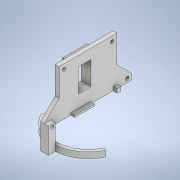
# Autodesk Inventor part: StaticGripper
Saved by Autodesk Inventor 2020 (Build 240168000, 168)
## iProperties
Created: 2023-01-18
Part Number: StaticGripper
Material: Generic
Document SubType Name: Modeling
Designer: legoo
Density: 1 g/cm^3
Appearance: Default
Author: legoo
## iProperties of the stored document _3DPrint.ipt
Created: 2023-01-18
Part Number: _3DPrint
Material: Generic
Document SubType Name: Modeling
Designer: legoo
Density: 1 g/cm^3
Appearance: Default
Author: legoo
Autodesk Inventor part; units mm, degrees
ref_plane "YZ Plane" through (0, 0, 0) normal (1, 0, 0) x (0, 1, 0)
ref_plane "XZ Plane" through (0, 0, 0) normal (0, 1, 0) x (-1, 0, 0)
ref_plane "XY Plane" through (0, 0, 0) normal (0, 0, 1) x (1, 0, 0)
sketch "Sketch1" plane through (0, 0, 0) normal (0, 1, 0) x (-1, 0, 0)
  line L0 (32.6452, 15.2227) -> (29.9263, 13.9549)
  line L1 (-29.9263, 13.9549) -> (-32.6452, 15.2227)
  line L2 (36.02, 0) -> (-36.02, 0) construction
  arc A0 (29.9263, 13.9549) -> (-29.9263, 13.9549) centre (0, 0) ccw
  arc A1 (32.6452, 15.2227) -> (-32.6452, 15.2227) centre (0, 0) ccw
  dimension "d2" = 25
  dimension "d3" = 25
  constraints: 6 end point, 4 point on circle, 2 centre point, 1 coincident, 1 horizontal
  measures "d2" angle of L0 L2
  measures "d3" angle of L2 L1
extrude "Extrusion1" add sketch "Sketch1" along normal blind 6
sketch "Sketch2" plane through (0, 0, 0) normal (0, -1, 0) x (1, 0, 0)
  arc A0 (32.6452, 15.2227) -> (-32.6452, 15.2227) centre (0, 0) ccw projected
  line L0 (2, 35.9644) -> (2, 42.9644)
  line L1 (2, 42.9644) -> (-2, 42.9644)
  line L2 (-2, 42.9644) -> (-2, 35.9644)
  dimension "d6" = 2
  dimension "d7" = 2
  dimension "d8" = 7
  constraints: 6 end point, 2 perpendicular, 2 point on circle, 1 vertical
  measures "d6" distance from line of point (0, 0) L0
  measures "d7" distance from line of point (0, 0) L2
  measures "d8" distance of L0.start L0.end
extrude "Extrusion2" add sketch "Sketch2" against normal blind 26
sketch "Sketch3" plane through (-2, 0, 35.9644) normal (-1, 0, 0) x (0, 0, 1)
  line L0 (7, 0) -> (7, 26) projected
  line L1 (7, 20) -> (-82.04, 20)
  line L2 (-82.04, 20) -> (-82.04, 26)
  line L3 (-82.04, 26) -> (-67.04, 41)
  line L4 (-67.04, 41) -> (-67.04, 69)
  line L5 (-67.04, 69) -> (-8, 69)
  line L6 (-8, 69) -> (-8, 41)
  line L7 (-8, 41) -> (7, 26)
  line L8 (-40.52, 59) -> (-27.52, 59)
  line L9 (-27.52, 59) -> (-27.52, 35)
  line L10 (-27.52, 35) -> (-40.52, 35)
  line L11 (-40.52, 35) -> (-40.52, 59)
  line L12 (7, 0) -> (0, 0) projected
  point P0 (-35.9644, 0)
  dimension "d11" = 15
  dimension "d12" = 15
  dimension "d13" = 89.04
  dimension "d14" = 24
  dimension "d15" = 13
  dimension "d16" = 19.52
  dimension "d17" = 10
  dimension "d18" = 15
  dimension "d19" = 15
  dimension "d20" = 15
  dimension "d21" = 20
  dimension "d22" = 6
  constraints: 22 end point, 4 perpendicular, 3 parallel, 2 horizontal, 1 point on line
  measures "d11" horizontal distance of L6.end L0.end
  measures "d12" horizontal distance of L3.end L2.end
  measures "d13" distance between parallel lines of L2 L0
  measures "d14" distance of L8.end L9.end
  measures "d15" distance of L8.start L8.end
  measures "d16" distance between parallel lines of L6 L9
  measures "d17" distance between parallel lines of L8 L5
  measures "d18" distance between parallel lines of L1 L10
  measures "d19" horizontal distance of L2.end L3.end
  measures "d20" horizontal distance of L0.end L6.end
  measures "d21" distance between parallel lines of L12 L1
  measures "d22" distance of L1.end L2.end
extrude "Extrusion3" add sketch "Sketch3" along normal blind 4
sketch "Sketch4" plane through (-6, 0, 35.9644) normal (-1, 0, 0) x (0, 0, 1)
  line L0 (-40.52, 35) -> (-40.52, 59) projected
  line L1 (-27.52, 35) -> (-40.52, 35) projected
  line L2 (-27.52, 59) -> (-27.52, 35) projected
  line L3 (-40.52, 59) -> (-27.52, 59) projected
  line L4 (-46.52, 29) -> (-46.52, 65)
  line L5 (-46.52, 65) -> (-21.52, 65)
  line L6 (-21.52, 65) -> (-21.52, 29)
  line L7 (-21.52, 29) -> (-46.52, 29)
  point P0 (-35.9644, 0)
  dimension "d49" = 6
  constraints: 8 end point, 3 other
  measures "d49" distance between parallel lines of L0 L4
extrude "Extrusion4" add sketch "Sketch4" along normal blind 6
sketch "Sketch5" plane through (-2, 20, -46.0756) normal (0, -1, 0) x (1, 0, 0)
  line L0 (0, 82.04) -> (0, 89.04) projected
  line L1 (0, 82.04) -> (0, 89.04)
  line L2 (0, 89.04) -> (-4, 89.04) projected
  line L3 (0, 89.04) -> (-4, 89.04)
  line L4 (-4, 89.04) -> (-4, 81.54)
  line L5 (-4, 89.04) -> (-4, 74.04) projected
  arc A0 (0, 82.04) -> (-30.6452, 61.2983) centre (2, 46.0756) ccw projected
  point P0 (-4, 81.5923)
  constraints: 6 end point, 2 collinear, 1 midpoint
extrude "Extrusion5" add sketch "Sketch5" along normal up to surface (20 mm away)
sketch "Sketch6" plane through (-2, 0, 35.9644) normal (1, 0, 0) x (0, 0, -1)
  circle A0 centre (77.54, 24) radius 1.75
  circle A1 centre (62.04, 64) radius 1.75
  circle A2 centre (13, 64) radius 1.75
  line L0 (8, 69) -> (67.04, 69) projected
  line L1 (67.04, 69) -> (67.04, 41) projected
  line L2 (8, 41) -> (8, 69) projected
  line L3 (82.04, 20) -> (0, 20) projected
  line L4 (82.04, 26) -> (82.04, 20) projected
  point P0 (35.9644, 0)
  dimension "d36" = 3.5
  dimension "d37" = 3.5
  dimension "d38" = 3.5
  dimension "d40" = 5
  dimension "d41" = 5
  dimension "d42" = 5
  dimension "d43" = 5
  dimension "d44" = 4
  dimension "d45" = 4.5
  constraints: 3 centre point
  measures "d36" diameter of A1
  measures "d37" diameter of A2
  measures "d38" diameter of A0
  measures "d40" distance from line of A1.centre L0
  measures "d41" distance from line of L1 A1.centre
  measures "d42" distance from line of L2 A2.centre
  measures "d43" distance from line of A2.centre L0
  measures "d44" distance from line of L3 A0.centre
  measures "d45" distance from line of L4 A0.centre
extrude "Extrusion6" cut sketch "Sketch6" against normal blind 6
sketch "Sketch7" plane through (2, 0, 42.9644) normal (1, 0, 0) x (0, 0, -1)
  circle A0 centre (4, 23) radius 1.75
  line L0 (0, 0) -> (0, 26) projected
  line L1 (0, 26) -> (7, 26) projected
  point P0 (42.9644, 0)
  dimension "d50" = 3.5
  dimension "d51" = 4
  dimension "d52" = 3
  constraints: 1 centre point
  measures "d50" diameter of A0
  measures "d51" distance from line of L0 A0.centre
  measures "d52" distance from line of L1 A0.centre
extrude "Extrusion7" cut sketch "Sketch7" against normal through all
sketch "Sketch8" plane through (-2, 0, 35.9644) normal (1, 0, 0) x (0, 0, -1)
  line L0 (82.04, 20) -> (0, 20) projected
  line L1 (20, 22) -> (40, 22)
  line L2 (40, 22) -> (40, 20)
  line L3 (40, 20) -> (20, 20)
  line L4 (20, 20) -> (20, 22)
  line L5 (0, 6) -> (0, 26) projected
  line L6 (67.04, 20) -> (63.04, 20)
  line L7 (63.04, 20) -> (63.04, 24)
  line L8 (63.04, 24) -> (67.04, 24)
  line L9 (67.04, 24) -> (67.04, 20)
  line L10 (82.04, 26) -> (82.04, 20) projected
  point P0 (35.9644, 0)
  dimension "d55" = 2
  dimension "d56" = 20
  dimension "d57" = 20
  dimension "d60" = 4
  dimension "d61" = 4
  dimension "d62" = 15
  constraints: 16 end point, 4 parallel, 2 horizontal, 2 perpendicular, 2 point on line
  measures "d55" distance between parallel lines of L0 L1
  measures "d56" distance between parallel lines of L4 L2
  measures "d57" distance between parallel lines of L5 L4
  measures "d60" distance of L7.end L8.end
  measures "d61" distance of L8.end L6.start
  measures "d62" distance between parallel lines of L10 L9
extrude "Extrusion8" add sketch "Sketch8" along normal blind 4
sketch "Sketch10" plane through (-6, 0, 35.9644) normal (-1, 0, 0) x (0, 0, 1)
  circle A0 centre (-62.04, 64) radius 1.75 projected
  circle A1 centre (-13, 64) radius 1.75 projected
  circle A2 centre (-77.54, 24) radius 1.75 projected
  circle A3 centre (3, 23) radius 1.75 projected
  line L0 (-62.04, 60.8246) -> (-64.79, 62.4123)
  line L1 (-64.79, 62.4123) -> (-64.79, 65.5877)
  line L2 (-64.79, 65.5877) -> (-62.04, 67.1754)
  line L3 (-62.04, 67.1754) -> (-59.29, 65.5877)
  line L4 (-59.29, 65.5877) -> (-59.29, 62.4123)
  line L5 (-59.29, 62.4123) -> (-62.04, 60.8246)
  line L6 (-13, 60.8246) -> (-15.75, 62.4123)
  line L7 (-15.75, 62.4123) -> (-15.75, 65.5877)
  line L8 (-15.75, 65.5877) -> (-13, 67.1754)
  line L9 (-13, 67.1754) -> (-10.25, 65.5877)
  line L10 (-10.25, 65.5877) -> (-10.25, 62.4123)
  line L11 (-10.25, 62.4123) -> (-13, 60.8246)
  line L12 (-74.79, 25.5877) -> (-74.79, 22.4123)
  line L13 (-74.79, 22.4123) -> (-77.54, 20.8246)
  line L14 (-77.54, 20.8246) -> (-80.29, 22.4123)
  line L15 (-80.29, 22.4123) -> (-80.29, 25.5877)
  line L16 (-80.29, 25.5877) -> (-77.54, 27.1754)
  line L17 (-77.54, 27.1754) -> (-74.79, 25.5877)
  circle A4 centre (3, 23) radius 1.75 projected
  line L18 (0.25, 24.5877) -> (3, 26.1754)
  line L19 (3, 26.1754) -> (5.75, 24.5877)
  line L20 (5.75, 24.5877) -> (5.75, 21.4123)
  line L21 (5.75, 21.4123) -> (3, 19.8246)
  line L22 (3, 19.8246) -> (0.25, 21.4123)
  line L23 (0.25, 21.4123) -> (0.25, 24.5877)
  line L24 (-67.04, 69) -> (-67.04, 41) projected
  line L25 (-8, 41) -> (-8, 69) projected
  line L26 (7, 26) -> (7, 0) projected
  line L27 (-82.04, 26) -> (-82.04, 20) projected
  point P0 (-35.9644, 0)
  dimension "d63" = 5.5
  dimension "d64" = 5.5
  dimension "d65" = 5.5
  dimension "d66" = 5.5
  constraints: 48 end point, 4 coincident, 4 parallel, 52 other
  measures "d63" distance between parallel lines of L1 L4
  measures "d64" distance between parallel lines of L10 L7
  measures "d65" distance between parallel lines of L12 L15
  measures "d66" distance between parallel lines of L23 L20
extrude "Extrusion9" cut sketch "Sketch10" against normal blind 2 contours A3 | L0 L1 L2 L3 L4 L5 | L6 L7 L8 L9 L10 L11 | L12 L13 L14 L15 L16 L17 | L18 L19 L20 L21 L22 L23
sketch "Sketch11" plane through (-12, 0, 35.9644) normal (-1, 0, 0) x (0, 0, 1)
  circle A0 centre (-34.02, 32.5) radius 0.5
  circle A1 centre (-34.02, 61.5) radius 0.5
  line L0 (-40.52, 59) -> (-27.52, 59) projected
  line L1 (-27.52, 35) -> (-40.52, 35) projected
  line L2 (-21.52, 29) -> (-21.52, 65) projected
  point P0 (-35.9644, 0)
  dimension "d69" = 2.5
  dimension "d70" = 2.5
  dimension "d71" = 12.5
  dimension "d72" = 12.5
  dimension "d73" = 1
  dimension "d74" = 1
  constraints: 2 centre point
  measures "d69" distance from line of A1.centre L0
  measures "d70" distance from line of A0.centre L1
  measures "d71" distance from line of L2 A0.centre
  measures "d72" distance from line of L2 A1.centre
  measures "d73" diameter of A1
  measures "d74" diameter of A0
extrude "Extrusion10" cut sketch "Sketch11" against normal blind 4
equation "\"d3\" = d2"
equation "\"d7\" = d6"
equation "\"d12\" = d11"
equation "\"d20\" = d19"
equation "\"d37\" = d36"
equation "\"d38\" = d36"
body "Solid1"
